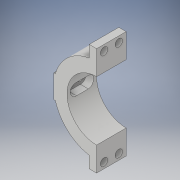
# Autodesk Inventor part: DremelHolder
Saved by Autodesk Inventor 2019 (Build 230136000, 136)
## iProperties
Created: 2019-05-13
Part Number: DremelHolder
Material: Generic
Document SubType Name: Modeling
Designer: Alex Jones
Density: 1 g/cm^3
Appearance: Default
Mass: 30.5642 g
Surface Area: 93.1195 cm^2
Volume: 30.5642 cm^3
Author: Alex Jones
Autodesk Inventor part; units mm, degrees
sketch "Sketch1" plane through (0, 0, 0) normal (0, 0, 1) x (1, 0, 0)
  arc A0 (-10, -8.75) -> (-8.75, -10) centre (-8.75, -8.75) ccw projected
  line L0 (-8.75, -10) -> (-3.6, -10) projected
  line L1 (-3.6, -10) -> (-3.1, -9.5) projected
  line L2 (-3.1, -9.5) -> (-3.1, -8.4) projected
  line L3 (-3.1, -8.4) -> (-5.5, -8.4) projected
  line L4 (-5.5, -8.4) -> (-5.5, -6.466) projected
  line L5 (-5.5, -6.466) -> (-3.134, -4.1) projected
  line L6 (-3.134, -4.1) -> (3.134, -4.1) projected
  line L7 (3.134, -4.1) -> (5.5, -6.466) projected
  line L8 (5.5, -6.466) -> (5.5, -8.4) projected
  line L9 (5.5, -8.4) -> (3.1, -8.4) projected
  line L10 (3.1, -8.4) -> (3.1, -9.5) projected
  line L11 (3.1, -9.5) -> (3.6, -10) projected
  line L12 (3.6, -10) -> (8.75, -10) projected
  arc A1 (8.75, -10) -> (10, -8.75) centre (8.75, -8.75) ccw projected
  line L13 (10, -8.75) -> (10, -3.6) projected
  line L14 (10, -3.6) -> (9.5, -3.1) projected
  line L15 (9.5, -3.1) -> (8.4, -3.1) projected
  line L16 (8.4, -3.1) -> (8.4, -5.5) projected
  line L17 (8.4, -5.5) -> (6.466, -5.5) projected
  line L18 (6.466, -5.5) -> (4.1, -3.134) projected
  line L19 (4.1, -3.134) -> (4.1, 3.134) projected
  line L20 (4.1, 3.134) -> (6.466, 5.5) projected
  line L21 (6.466, 5.5) -> (8.4, 5.5) projected
  line L22 (8.4, 5.5) -> (8.4, 3.1) projected
  line L23 (8.4, 3.1) -> (9.5, 3.1) projected
  line L24 (9.5, 3.1) -> (10, 3.6) projected
  line L25 (10, 3.6) -> (10, 8.75) projected
  arc A2 (10, 8.75) -> (8.75, 10) centre (8.75, 8.75) ccw projected
  line L26 (8.75, 10) -> (3.6, 10) projected
  line L27 (3.6, 10) -> (3.1, 9.5) projected
  line L28 (3.1, 9.5) -> (3.1, 8.4) projected
  line L29 (3.1, 8.4) -> (5.5, 8.4) projected
  line L30 (5.5, 8.4) -> (5.5, 6.466) projected
  line L31 (5.5, 6.466) -> (3.134, 4.1) projected
  line L32 (3.134, 4.1) -> (-3.134, 4.1) projected
  line L33 (-3.134, 4.1) -> (-5.5, 6.466) projected
  line L34 (-5.5, 6.466) -> (-5.5, 8.4) projected
  line L35 (-5.5, 8.4) -> (-3.1, 8.4) projected
  line L36 (-3.1, 8.4) -> (-3.1, 9.5) projected
  line L37 (-3.1, 9.5) -> (-3.6, 10) projected
  line L38 (-3.6, 10) -> (-8.75, 10) projected
  arc A3 (-8.75, 10) -> (-10, 8.75) centre (-8.75, 8.75) ccw projected
  line L39 (-10, 8.75) -> (-10, 3.6) projected
  line L40 (-10, 3.6) -> (-9.5, 3.1) projected
  line L41 (-9.5, 3.1) -> (-8.4, 3.1) projected
  line L42 (-8.4, 3.1) -> (-8.4, 5.5) projected
  line L43 (-8.4, 5.5) -> (-6.466, 5.5) projected
  line L44 (-6.466, 5.5) -> (-4.1, 3.134) projected
  line L45 (-4.1, 3.134) -> (-4.1, -3.134) projected
  line L46 (-4.1, -3.134) -> (-6.466, -5.5) projected
  line L47 (-6.466, -5.5) -> (-8.4, -5.5) projected
  line L48 (-8.4, -5.5) -> (-8.4, -3.1) projected
  line L49 (-8.4, -3.1) -> (-9.5, -3.1) projected
  line L50 (-9.5, -3.1) -> (-10, -3.6) projected
  line L51 (-10, -3.6) -> (-10, -8.75) projected
  circle A4 centre (0, 0) radius 2.5 projected
  circle A5 centre (46.7, 0) radius 4.5 projected
  arc A6 (46.7103, 25.4) -> (46.7103, -25.4) centre (46.7, 0) ccw
  line L52 (10, 10) -> (16.35, 10)
  line L53 (16.35, 10) -> (16.35, -10)
  line L54 (16.35, -10) -> (10, -10)
  line L55 (10, -10) -> (10, 10)
  arc A7 (46.7103, 36.7) -> (46.7103, -36.7) centre (46.7, 0) ccw
  line L56 (46.7103, 36.7) -> (46.7103, 25.4)
  line L57 (46.7103, -25.4) -> (46.7103, -36.7)
  dimension "d0" = 50.8
  dimension "d1" = 20
  dimension "d2" = 6.35
  constraints: 12 end point, 4 point on circle, 2 centre point, 2 coincident, 2 parallel, 1 horizontal, 1 perpendicular, 1 point on line, 1 tangent
  measures "d0" diameter of A6
  measures "d1" distance of L54.end L52.start
  measures "d2" distance of L53.end L54.end
extrude "Extrusion1" add sketch "Sketch1" along normal blind 25.4 contours L13 L55 A7 L54 | L55 L25 L52 A7 | A7 L52 L53 L54 | L54 L53 L52 A7 L56 A6 L57
ref_plane "Work Plane1" through (46.7103, 36.7, 0) normal (0, 1, 0) x (0, 0, 1)
sketch "Sketch2" plane through (46.7103, 36.7, 0) normal (0, 1, 0) x (0, 0, 1)
  line L0 (0, 0) -> (25.4, 0) projected
  line L1 (25.4, -35.3216) -> (25.4, 0) projected
  line L2 (0, 0) -> (25.4, 0)
  line L3 (25.4, 0) -> (25.4, -6.35)
  line L4 (25.4, -6.35) -> (0, -6.35)
  line L5 (0, -6.35) -> (0, 0)
  point P0 (0, -46.7103)
  dimension "d6" = 6.35
  constraints: 8 end point, 2 parallel, 1 horizontal, 1 perpendicular, 1 point on line
  measures "d6" distance between parallel lines of L4 L0
extrude "Extrusion2" add sketch "Sketch2" along normal mid plane 19.05
ref_plane "Work Plane2" through (10, 0, 0) normal (0, 1, 0) x (1, 0, 0)
mirror "Mirror1" about plane through (10, 0, 0) normal (0, 1, 0) of "Extrusion2"
sketch "Sketch3" plane through (46.7103, -25.4, 25.4) normal (1, 0, 0) x (0, 0, -1)
  circle A0 centre (19.05, -15.7382) radius 3.175 projected
  circle A1 centre (6.35, -15.7382) radius 3.175 projected
  circle A2 centre (6.35, 66.5382) radius 3.175 projected
  circle A3 centre (19.05, 66.5382) radius 3.175 projected
  point P0 (25.4, 25.4)
extrude "Extrusion3" cut sketch "Sketch3" against normal through all
ref_plane "Work Plane4" through (21.3, 0, 0) normal (-1, 0, 0) x (0, -1, 0)
ref_plane "Work Plane3" through (72.1, 0, 0) normal (-1, 0, 0) x (0, -1, 0)
sketch "Sketch4" plane through (72.1, 0, 0) normal (-1, 0, 0) x (0, -1, 0)
  line L0 (0, 0) -> (0, 25.4) construction
  line L1 (-10, 25.4) -> (10, 25.4) projected
  circle A0 centre (0, 17.78) radius 2.75
  circle A1 centre (0, 7.62) radius 2.75
  line L2 (-25.4, 0) -> (25.4, 0) projected
  dimension "d13" = 5.5
  dimension "d14" = 7.62
  dimension "d15" = 7.62
  constraints: 2 centre point, 2 end point, 2 point on line, 1 equal radius, 1 midpoint
  measures "d13" diameter of A0
  measures "d14" distance from line of L1 A0.centre
  measures "d15" distance from line of L2 A1.centre
extrude "Extrusion4" cut sketch "Sketch4" along normal through all
sketch "Sketch5" plane through (72.1, 0, 0) normal (-1, 0, 0) x (0, -1, 0)
  spline S0 degree 2 poles (2.75, 17.78) (2.75, 13.0169) (-1.375, 15.3984) (-5.5, 17.78) (-1.375, 20.1616) (2.75, 22.5431) (2.75, 17.78) knots 0 0 0 0.333333 0.333333 0.666667 0.666667 1 1 1 weights 1 0.5 1 0.5 1 0.5 1 projected
  spline S1 degree 2 poles (2.75, 7.62) (2.75, 2.8569) (-1.375, 5.2384) (-5.5, 7.62) (-1.375, 10.0016) (2.75, 12.3831) (2.75, 7.62) knots 0 0 0 0.333333 0.333333 0.666667 0.666667 1 1 1 weights 1 0.5 1 0.5 1 0.5 1 projected
  circle A0 centre (0, 7.62) radius 2.75 projected
  line L0 (5, 12.7) -> (5, 7.62)
  arc A1 (-5, 7.62) -> (5, 7.62) centre (0, 7.62) ccw
  spline S2 degree 7 poles (2.75, 17.78) (2.75, 18.0802) (2.7118, 18.38) (2.6355, 18.6767) (2.52, 18.9674) (2.3634, 19.248) (2.1631, 19.5126) (1.7177, 19.9454) (1.4837, 20.1274) (1.2158, 20.2864) (0.9183, 20.4129) (0.5978, 20.4988) (0.2624, 20.5386) (-0.4242, 20.519) (-0.7584, 20.4587) (-1.0728, 20.3535) (-1.3607, 20.2102) (-1.617, 20.0371) (-1.8389, 19.8434) (-2.2394, 19.407) (-2.4132, 19.1552) (-2.5494, 18.8907) (-2.6501, 18.6181) (-2.7166, 18.3405) (-2.75, 18.0604) (-2.75, 17.4798) (-2.7118, 17.18) (-2.6355, 16.8833) (-2.52, 16.5926) (-2.3634, 16.312) (-2.1631, 16.0474) (-1.7177, 15.6146) (-1.4837, 15.4326) (-1.2158, 15.2736) (-0.9183, 15.1471) (-0.5978, 15.0612) (-0.2624, 15.0214) (0.4242, 15.041) (0.7584, 15.1013) (1.0728, 15.2065) (1.3607, 15.3498) (1.617, 15.5229) (1.8389, 15.7166) (2.2394, 16.153) (2.4132, 16.4048) (2.5494, 16.6693) (2.6501, 16.9419) (2.7166, 17.2195) (2.75, 17.4996) (2.75, 17.78) knots 0 0 0 0 0 0 0 0 0.14065 0.14065 0.14065 0.14065 0.14065 0.14065 0.254122 0.254122 0.254122 0.254122 0.254122 0.254122 0.369156 0.369156 0.369156 0.369156 0.369156 0.369156 0.500342 0.500342 0.500342 0.500342 0.500342 0.500342 0.640802 0.640802 0.640802 0.640802 0.640802 0.640802 0.754121 0.754121 0.754121 0.754121 0.754121 0.754121 0.869 0.869 0.869 0.869 0.869 0.869 1 1 1 1 1 1 1 1 projected
  line L1 (25.4, 0) -> (-25.4, 0) projected
  line L2 (-25.4, 0) -> (-25.4, 25.4) projected
  line L3 (25.4, 25.4) -> (-25.4, 25.4) projected
  line L4 (25.4, 0) -> (25.4, 25.4) projected
  line L5 (-10, 25.4) -> (10, 25.4) projected
  line L6 (0, 25.4) -> (0, 20.53)
  line L7 (0, 15.03) -> (0, 10.37) construction
  line L8 (0, 4.87) -> (0, 0)
  line L9 (-5.6857, 12.7) -> (9.2801, 12.7) construction
  line L10 (-5, 7.62) -> (-5, 12.7)
  line L11 (5, 12.7) -> (5, 17.78)
  arc A2 (5, 17.78) -> (-5, 17.78) centre (0, 17.78) ccw
  line L12 (-5, 17.78) -> (-5, 12.7)
  constraints: 16 end point, 7 point on circle, 4 point on line, 4 symmetric about line, 4 vertical, 2 centre point, 1 coincident, 1 horizontal, 1 midpoint, 1 perpendicular, 8 other
extrude "Extrusion5" cut sketch "Sketch5" along normal blind 57.15 contours L0 A1 L10 L12 A2 L11
body "Solid1"
